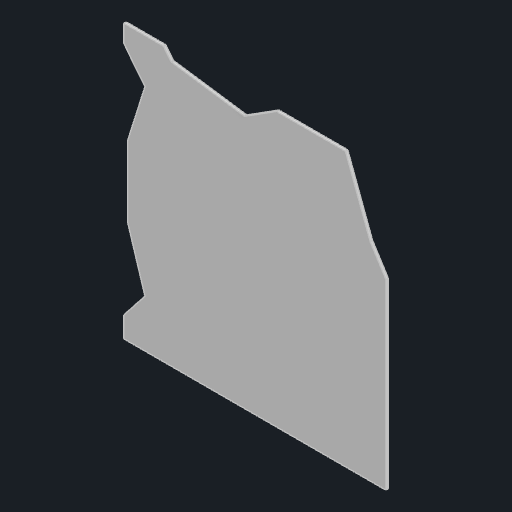
# Autodesk Inventor part: ChestTopPanel
Saved by Autodesk Inventor 2025.2 (Build 292293000, 293)
## iProperties
Created: 2025-10-05
Part Number: ChestTopPanel
Material: Generic
Document SubType Name: Sheet Metal
Designer: valer
Density: 1 g/cm^3
Sheet Metal Rule: Default
Appearance: Default
Author: valer
Autodesk Inventor part; units mm, degrees
ref_plane "YZ Plane" through (0, 0, 0) normal (1, 0, 0) x (0, 1, 0)
ref_plane "XZ Plane" through (0, 0, 0) normal (0, 1, 0) x (-1, 0, 0)
ref_plane "XY Plane" through (0, 0, 0) normal (0, 0, 1) x (1, 0, 0)
sketch "Base" plane through (0, 0, 0) normal (0, 0, 1) x (1, 0, 0)
  line L0 (370.5814, -184.5855) -> (20.5814, -184.5855)
  line L1 (20.5814, -184.5855) -> (20.5814, 180.4145)
  line L2 (20.5814, 180.4145) -> (370.5814, 180.4145)
  line L3 (370.5814, 180.4145) -> (370.5814, -184.5855)
  point P0 (0, 0)
  dimension "d1" = 365
  dimension "d3" = 350
  measures "d1" distance of L2.end L0.start
  measures "d3" distance of L0.start L0.end
extrude "Plate1" add sketch "Base" along normal blind 3.048
sketch "Sketch3" plane through (0, 0, 0) normal (0, 0, -1) x (-1, 0, 0)
  line L0 (-20.5814, 180.4145) -> (-20.5814, -184.5855) projected
  line L1 (-20.5814, 157.0475) -> (-48.8438, 121.1909)
  line L2 (-48.8438, 121.1909) -> (-25.7113, 47.3877)
  line L3 (-25.7113, 0) -> (-25.7113, 47.3877)
  line L4 (-370.5814, -184.5855) -> (-370.5814, 180.4145) projected
  line L5 (-370.5814, 180.4145) -> (-20.5814, 180.4145) projected
  line L6 (-73.6607, 180.4145) -> (-83.9743, 167.3295)
  line L7 (-83.9743, 167.3295) -> (-181.8072, 153.3458)
  line L8 (-181.8072, 153.3458) -> (-224.5475, 180.4145)
  line L9 (-316.5549, 180.4145) -> (-349.6972, 92.1919)
  line L10 (-349.6972, 92.1919) -> (-370.5814, 59.2166)
  line L11 (49.4186, 0) -> (-440.5814, 0) construction
  line L12 (-20.5814, -157.0475) -> (-48.8438, -121.1909)
  line L13 (-25.7113, 0) -> (-25.7113, -47.3877)
  line L14 (-73.6607, -180.4145) -> (-83.9743, -167.3295)
  line L15 (-83.9743, -167.3295) -> (-181.8072, -153.3458)
  line L16 (-181.8072, -153.3458) -> (-224.5475, -180.4145)
  line L17 (-316.5549, -180.4145) -> (-349.6972, -92.1919)
  line L18 (-349.6972, -92.1919) -> (-370.5814, -59.2166)
  line L19 (-25.7113, -47.3877) -> (-48.8438, -121.1909)
  constraints: 32 end point, 10 symmetric about line, 6 point on line
extrude "Cut1" cut sketch "Sketch3" against normal blind 3.048
equation "\"d5\" = Thickness"
equation "\"d4\" = Thickness"
equation "\"BendRadius\" = Thickness"
equation "\"BendReliefWidth\" = Thickness"
equation "\"BendReliefDepth\" = 0.5 * Thickness"
equation "\"CornerReliefSize\" = 4 * Thickness"
equation "\"MinimumRemnant\" = 2 * Thickness"
equation "\"TransitionRadius\" = BendRadius"
equation "\"JacobiRadiusSize\" = BendRadius"
equation "\"GapSize\" = Thickness"
equation "\"Thickness\" = 3.048"
body "Solid1"
